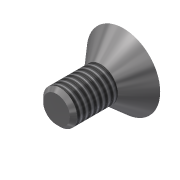
# Autodesk Inventor part: 10-32 Flathead x375
Saved by Autodesk Inventor 2013 (Build 170138000, 138)
## iProperties
Created: 2014-02-02
Part Number: 10-32 Flathead x375
Material: Steel, Alloy
Document SubType Name: Modeling
Designer: Nemo
Density: 1 g/cm^3
Author: Nemo
Autodesk Inventor part; units mm, degrees
ref_plane "YZ Plane" through (0, 0, 0) normal (1, 0, 0) x (0, 1, 0)
ref_plane "XZ Plane" through (0, 0, 0) normal (0, 1, 0) x (-1, 0, 0)
ref_plane "XY Plane" through (0, 0, 0) normal (0, 0, 1) x (1, 0, 0)
sketch "Sketch1" plane through (0, 0, 0) normal (0, 1, 0) x (-1, 0, 0)
  line L0 (0, 0) -> (0, 9.525)
  line L1 (0, 9.525) -> (-2.413, 9.525)
  line L2 (-2.413, 9.525) -> (-2.413, 3.2258)
  line L3 (-2.413, 3.2258) -> (-5.2171, 0)
  line L4 (-5.2171, 0) -> (0, 0)
  dimension "d0" = 4.826
  dimension "d2" = 9.525
  dimension "d3" = 41
  dimension "d4" = 3.2258
  dimension "d5" = 5.2172
  constraints: 10 end point, 2 parallel, 1 perpendicular, 1 vertical
  measures "d0" diameter of L2 L0
  measures "d2" distance between parallel lines of L1 L4
  measures "d3" angle of L0 L3
  measures "d4" distance from line of L2.end L4
  measures "d5" distance of L3.end L0.start
revolve "Revolution1" add sketch "Sketch1" angle 360 about axis through (0, 0, 0) along (0, 0, 1)
thread "Thread1" size "10-32 UNF" class "2A" standard "ANSI Unified Screw Threads" full length
chamfer "Chamfer1" distance 0.508 angle 45 1 edges at (-2.413, 0, 9.525)
sketch "Sketch2" plane through (0, 0, 0) normal (0, 0, -1) x (-1, 0, 0)
  circle A0 centre (0, 0) radius 5.2171 projected
  line L0 (0.9165, -1.5875) -> (-0.9165, -1.5875)
  line L1 (-0.9165, -1.5875) -> (-1.8331, 0)
  line L2 (-1.8331, 0) -> (-0.9165, 1.5875)
  line L3 (-0.9165, 1.5875) -> (0.9165, 1.5875)
  line L4 (0.9165, 1.5875) -> (1.8331, 0)
  line L5 (1.8331, 0) -> (0.9165, -1.5875)
  dimension "d12" = 3.175
  constraints: 12 end point, 1 coincident, 1 horizontal, 13 other
  measures "d12" distance between parallel lines of L0 L3
extrude "Extrusion1" cut sketch "Sketch2" against normal blind 2.032 contours L0 L1 L2 L3 L4 L5
body "Solid1"
